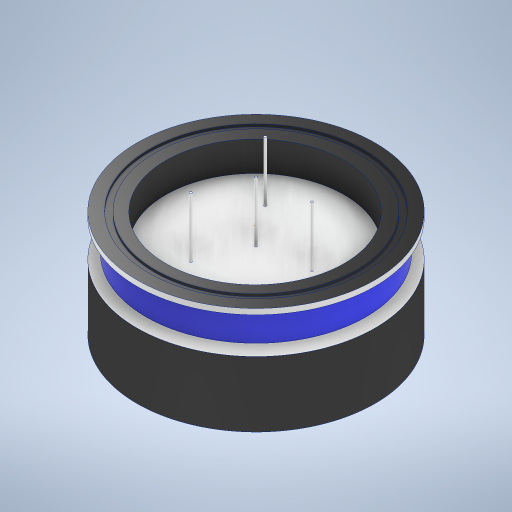
# Autodesk Inventor part: Base
Saved by Autodesk Inventor 2024 (Build 280153000, 153)
## iProperties
Created: 2023-07-08
Part Number: Base
Material: Generic
Document SubType Name: Modeling
Designer: westy
Density: 1 g/cm^3
Appearance: Aluminum - Flat
Author: westy
Autodesk Inventor part; units mm, degrees
ref_plane "YZ Plane" through (0, 0, 0) normal (1, 0, 0) x (0, 1, 0)
ref_plane "XZ Plane" through (0, 0, 0) normal (0, 1, 0) x (-1, 0, 0)
ref_plane "XY Plane" through (0, 0, 0) normal (0, 0, 1) x (1, 0, 0)
sketch "Sketch1" plane through (0, 0, 0) normal (0, 1, 0) x (-1, 0, 0)
  circle A0 centre (0, 0) radius 100
  circle A1 centre (0, 0) radius 90
  circle A2 centre (0, 0) radius 85
  dimension "d0" = 200
  dimension "d1" = 180
  dimension "d2" = 170
  constraints: 3 centre point, 3 coincident
  measures "d0" diameter of A0
  measures "d1" diameter of A1
  measures "d2" diameter of A2
extrude "Extrusion1" add sketch "Sketch1" along normal blind 8 contours A0 | A1 | A2
extrude "Extrusion2" add sketch "Sketch1" along normal blind 10
extrude "Extrusion3" add sketch "Sketch1" against normal blind 80 contours A0 | A1 | A2
sketch "Sketch2" plane through (0, 10, 0) normal (0, 1, 0) x (1, 0, 0)
  circle A0 centre (0, -0.8314) radius 75
  point P0 (0, 0)
  dimension "d9" = 150
  constraints: 1 centre point
  measures "d9" diameter of A0
extrude "Extrusion4" cut sketch "Sketch2" against normal blind 25
sketch "Sketch3" plane through (0, 0, 0) normal (1, 0, 0) x (0, 1, 0)
  line L0 (5.4504, 100.114) -> (0.3612, 91.2991)
  line L1 (5.4504, 100.114) -> (15.629, 100.114) construction
  line L2 (-80, 100) -> (10, 100) projected
  line L3 (-25, 100) -> (-20.6699, 92.5)
  line L4 (-25, 100) -> (-16.3397, 100) construction
  line L5 (-20.6699, 92.5) -> (1.0545, 92.5)
  line L6 (5.4504, 100.114) -> (-20.6699, 100)
  line L7 (-33.1258, 0) -> (23.7548, 0) projected
  line L8 (1.0545, 92.5) -> (-70.8596, 92.5)
  line L9 (-70.8596, 92.5) -> (-80, 100)
  point P0 (0, 0)
  point P1 (5.3846, 100)
  dimension "d12" = 120
  dimension "d13" = 60
  constraints: 16 end point, 3 horizontal, 3 point on line, 2 equal length, 1 midpoint
  measures "d12" angle of L0 L1
  measures "d13" angle of L3 L4
revolve "Revolution1" cut sketch "Sketch3" angle 360 about axis through (0, -10, 0) along (0, 1, 0) contours L0 L5 L3 L2
sketch "Sketch6" plane through (0, -15, 0.8314) normal (0, 1, 0) x (1, 0, 0)
  circle A0 centre (0, 0.8314) radius 42
  circle A1 centre (-25.5623, 34.1567) radius 1
  circle A2 centre (-16.0794, -37.9688) radius 1
  circle A3 centre (41.6416, 6.3064) radius 1
  circle A4 centre (0, 0.8314) radius 1
  dimension "d32" = 84
  dimension "d33" = 2
  dimension "d36" = 360
  dimension "d40" = 2
  constraints: 4 centre point, 2 coincident, 10 other
  measures "d33" diameter of A1
  measures "d40" diameter of A4
extrude "Extrusion7" add sketch "Sketch6" along normal blind 50 contours A3 A0 | A0 A3 | A2 A0 | A0 A2 | A1 A0 | A0 A1 | A4
body "Solid1"
